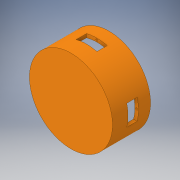
# Autodesk Inventor part: Base
Saved by Autodesk Inventor 2019 (Build 230136000, 136)
## iProperties
Created: 2022-07-05
Part Number: Base
Material: Generic
Document SubType Name: Modeling
Designer: zreik
Density: 1 g/cm^3
Appearance: Orange
Author: zreik
Autodesk Inventor part; units mm, degrees
ref_plane "YZ Plane" through (0, 0, 0) normal (1, 0, 0) x (0, 1, 0)
ref_plane "XZ Plane" through (0, 0, 0) normal (0, 1, 0) x (-1, 0, 0)
ref_plane "XY Plane" through (0, 0, 0) normal (0, 0, 1) x (1, 0, 0)
sketch "Sketch1" plane through (0, 0, 0) normal (0, 0, 1) x (1, 0, 0)
  circle A0 centre (0, 0) radius 60
  circle A1 centre (0, 0) radius 55
  circle A2 centre (0, 57.5) radius 1.5
  circle A3 centre (-57.5, 0) radius 1.5
  circle A4 centre (0, -57.5) radius 1.5
  circle A5 centre (57.5, 0) radius 1.5
  dimension "d2" = 120
  dimension "d3" = 110
  dimension "d4" = 3
  dimension "d5" = 0
  dimension "d6" = 57.5
  dimension "d7" = 360
  constraints: 6 centre point, 3 coincident, 9 other
  measures "d2" diameter of A0
  measures "d3" diameter of A1
  measures "d4" diameter of A2
  measures "d5" horizontal distance of point (0, 0) A2.centre
  measures "d6" distance of point (0, 0) A2.centre
extrude "Extrusion1" add sketch "Sketch1" along normal blind 5 contours A0 | A1
extrude "Extrusion2" add sketch "Sketch1" against normal blind 50
extrude "Extrusion3" add sketch "Sketch1" along normal mid plane 10 contours A2 | A3 | A4 | A5
sketch "Sketch2" plane through (0, 0, 0) normal (0, 1, 0) x (-1, 0, 0)
  line L0 (-15, -17.5) -> (15, -17.5)
  line L1 (15, -17.5) -> (15, -32.5)
  line L2 (15, -32.5) -> (-15, -32.5)
  line L3 (-15, -32.5) -> (-15, -17.5)
  line L4 (-15, -17.5) -> (15, -32.5) construction
  line L5 (15, -17.5) -> (-15, -32.5) construction
  point P0 (0, 0)
  point P1 (0, -25)
  dimension "d14" = 0
  dimension "d15" = 25
  dimension "d16" = 30
  dimension "d17" = 15
  constraints: 12 end point, 2 midpoint, 2 parallel, 1 horizontal, 1 perpendicular
  measures "d14" horizontal distance of point (0, 0) point (0, -25)
  measures "d15" distance of point (0, 0) point (0, -25)
  measures "d16" distance of L1.end L2.end
  measures "d17" distance of L0.end L1.end
extrude "Extrusion4" cut sketch "Sketch2" along normal through all both and the other way through all
pattern_circular "Circular Pattern1" count 3 over 180 about axis through (0, 0, 0) along (0, 0, -1) of "Extrusion4"
extrude "Extrusion5" add sketch "Sketch1" against normal blind 17.5 contours A2 | A3 | A4 | A5
equation "\"d2\" = Diameter"
equation "\"d6\" = 0.25 * d2 + 0.25 * d3"
equation "\"Diameter\" = 120"
body "Solid1"
